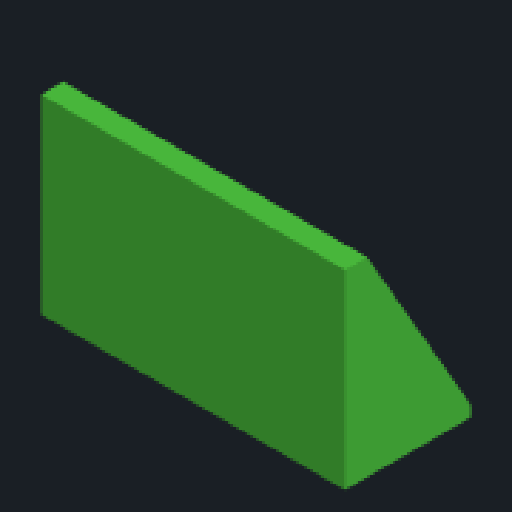
# Autodesk Inventor part: case1
Saved by Autodesk Inventor 2026.2 (Build 302298000, 298)
## iProperties
Created: 2026-01-27
Part Number: case1
Material: Generic
Document SubType Name: Modeling
Designer: test
Density: 1 g/cm^3
Appearance: Default
Author: test
## iProperties of the stored document case1_3DPrint.ipt
Created: 2026-01-27
Part Number: case1_3DPrint
Material: Generic
Document SubType Name: Modeling
Designer: test
Density: 1 g/cm^3
Appearance: Default
Author: test
Autodesk Inventor part; units mm, degrees
ref_plane "YZ Plane" through (0, 0, 0) normal (1, 0, 0) x (0, 1, 0)
ref_plane "XZ Plane" through (0, 0, 0) normal (0, 1, 0) x (-1, 0, 0)
ref_plane "XY Plane" through (0, 0, 0) normal (0, 0, 1) x (1, 0, 0)
sketch "Sketch1" plane through (0, 0, 0) normal (1, 0, 0) x (0, 1, 0)
  line L0 (0, 0) -> (171.9468, 0)
  line L1 (171.9468, 0) -> (171.9468, -20)
  line L2 (171.9468, -20) -> (10, -113.5)
  line L3 (10, -113.5) -> (0, -113.5)
  line L4 (0, -113.5) -> (0, 0)
  dimension "d0" = 187
  dimension "d1" = 60
  dimension "d2" = 10
  dimension "d3" = 20
  constraints: 10 end point, 2 perpendicular, 1 horizontal, 1 parallel
  measures "d0" distance of L1.end L2.end
  measures "d1" angle of L4 L2
  measures "d2" distance of L2.end L3.end
  measures "d3" distance of L0.end L1.end
extrude "Extrusion1" add sketch "Sketch1" along normal blind 274.11
body "Solid1"
